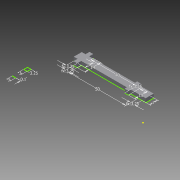
# Autodesk Inventor part: body-back
Saved by Autodesk Inventor 2013 (Build 170138000, 138)
## iProperties
Created: 2012-09-08
Part Number: body-back
Material: Generic
Document SubType Name: Modeling
Designer: frankenteddy
Density: 1 g/cm^3
Author: frankenteddy
Autodesk Inventor part; units mm, degrees
ref_plane "YZ Plane" through (0, 0, 0) normal (1, 0, 0) x (0, 1, 0)
ref_plane "XZ Plane" through (0, 0, 0) normal (0, 1, 0) x (-1, 0, 0)
ref_plane "XY Plane" through (0, 0, 0) normal (0, 0, 1) x (1, 0, 0)
sketch "Sketch1" plane through (0, 0, 0) normal (0, 0, 1) x (1, 0, 0)
  line L0 (-92.7646, -8.503) -> (-89.7646, -8.503)
  line L1 (-89.7646, -8.503) -> (-89.7646, -11.753)
  line L2 (-89.7646, -11.753) -> (-92.7646, -11.753)
  line L3 (-92.7646, -11.753) -> (-92.7646, -8.503)
  line L4 (-92.7646, -21.6527) -> (-89.7646, -21.6527)
  line L5 (-89.7646, -21.6527) -> (-89.7646, -21.7527)
  line L6 (-89.7646, -21.7527) -> (-92.7646, -21.7527)
  line L7 (-92.7646, -21.7527) -> (-92.7646, -21.6527)
  line L8 (-70.621, 23.5389) -> (-20.621, 23.5389)
  line L9 (-20.621, 23.5389) -> (-20.621, 16.5389)
  line L10 (-20.621, 16.5389) -> (-70.621, 16.5389)
  line L11 (-70.621, 16.5389) -> (-70.621, 23.5389)
  line L12 (-73.871, 27.0389) -> (-70.621, 27.0389)
  line L13 (-70.621, 27.0389) -> (-70.621, 13.0389)
  line L14 (-70.621, 13.0389) -> (-73.871, 13.0389)
  line L15 (-73.871, 13.0389) -> (-73.871, 27.0389)
  line L16 (-73.871, 20.0389) -> (-70.621, 20.0389) construction
  line L17 (-20.621, 20.0389) -> (-70.621, 20.0389) construction
  line L18 (-45.621, 23.5389) -> (-45.621, 16.5389) construction
  line L19 (-77.121, 23.5389) -> (-73.871, 23.5389)
  line L20 (-73.871, 23.5389) -> (-73.871, 16.5389)
  line L21 (-73.871, 16.5389) -> (-77.121, 16.5389)
  line L22 (-77.121, 16.5389) -> (-77.121, 23.5389)
  line L23 (-77.121, 20.0389) -> (-73.871, 20.0389) construction
  line L24 (-20.621, 23.5389) -> (-17.371, 23.5389)
  line L25 (-17.371, 23.5389) -> (-17.371, 16.5389)
  line L26 (-17.371, 16.5389) -> (-20.621, 16.5389)
  line L27 (-20.621, 16.5389) -> (-20.621, 23.5389)
  line L28 (-14.121, 23.5389) -> (-17.371, 23.5389)
  line L29 (-17.371, 23.5389) -> (-17.371, 16.5389)
  line L30 (-17.371, 16.5389) -> (-14.121, 16.5389)
  line L31 (-14.121, 16.5389) -> (-14.121, 23.5389)
  line L32 (-14.121, 20.0389) -> (-17.371, 20.0389) construction
  line L33 (-30.621, 25.5389) -> (-27.371, 25.5389)
  line L34 (-27.371, 25.5389) -> (-27.371, 14.5389)
  line L35 (-27.371, 14.5389) -> (-30.621, 14.5389)
  line L36 (-30.621, 14.5389) -> (-30.621, 25.5389)
  line L37 (-30.621, 20.0389) -> (-27.371, 20.0389) construction
  point P0 (0, 0)
  point P1 (-17.371, 20.0389)
  dimension "d3" = 3
  dimension "mat" = 3.25
  dimension "d5" = 3
  dimension "kerf" = 0.1
  dimension "d44" = 3.25
  dimension "d45" = 14
  dimension "d46" = 3.25
  dimension "d47" = 7
  dimension "d48" = 50
  dimension "d49" = 3.25
  dimension "d50" = 7
  dimension "d53" = 3.25
  dimension "d54" = 11
  dimension "d55" = 40
  constraints: 76 end point, 14 parallel, 10 midpoint, 8 collinear, 8 perpendicular, 7 horizontal, 5 symmetric about line
  measures "d3" distance of L1.end L2.end
  measures "mat" distance of L0.end L1.end
  measures "d5" distance of L5.end L6.end
  measures "kerf" distance of L4.end L5.end
  measures "d44" distance of L13.end L14.end
  measures "d45" distance of L12.end L13.end
  measures "d46" distance of L20.end L21.end
  measures "d47" distance of L19.end L20.end
  measures "d48" distance of L9.end L10.end
  measures "d49" distance of L25.end L26.end
  measures "d50" distance of L24.end L25.end
  measures "d53" distance of L34.end L35.end
  measures "d54" distance of L33.end L34.end
  measures "d55" distance between parallel lines of L36 L13
extrude "Extrusion6" add sketch "Sketch1" along normal blind 3.25 contours L8 L36 L10 L11 | L11 L13 L14 L15 L12 | L8 L34 L10 L36 | L8 L9 L10 L34 | L24 L25 L26 L9 | L15 L21 L22 L19 | L28 L31 L30 L25
extrude "Extrusion7" add sketch "Sketch1" along normal blind 3.25 contours L36 L33 L34 L8 | L8 L34 L10 L36 | L10 L34 L35 L36
equation "\"d44\" = mat"
equation "\"d46\" = mat"
equation "\"d49\" = mat"
equation "\"d53\" = mat"
equation "\"d51\" = mat"
equation "\"d56\" = mat"
body "Solid3"
